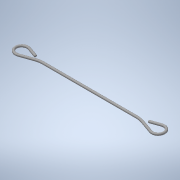
# Autodesk Inventor part: Rebar type 1
Saved by Autodesk Inventor 2021 (Build 250183000, 183)
## iProperties
Company: SDU
Created: 2020-10-29
Part Number: Rebar type 1
Engr Approved By: Approved By
Material: Steel
Description: Description
Document SubType Name: Modeling
Designer: Kling
Engineer: Engineer
Stock Number: Stock number
Density: 7.85 g/cm^3
Appearance: Steel
RM. Dwg. No.: 5674
RM. File Name: N.A.
RM. No.: 4789
Title: Title
Author: Kling
Autodesk Inventor part; units mm, degrees
ref_plane "YZ Plane" through (0, 0, 0) normal (1, 0, 0) x (0, 1, 0)
ref_plane "XZ Plane" through (0, 0, 0) normal (0, 1, 0) x (-1, 0, 0)
ref_plane "XY Plane" through (0, 0, 0) normal (0, 0, 1) x (1, 0, 0)
sketch "Sketch1" plane through (0, 0, 0) normal (0, 0, 1) x (1, 0, 0)
  line L0 (0, 0) -> (-79.8528, 0)
  line L1 (-89.8528, -1.7157) -> (-111.6667, -9.4281)
  arc A0 (-111.6667, 9.4281) -> (-111.6667, -9.4281) centre (-115, 0) ccw
  line L2 (-111.6667, 9.4281) -> (-94.8528, 3.4835)
  arc A1 (-79.8528, 0) -> (-89.8528, -1.7157) centre (-79.8528, -30) ccw
  line L3 (0, 0) -> (0, 44.256) construction
  line L4 (0, 0) -> (79.8528, 0)
  line L5 (89.8528, -1.7157) -> (111.6667, -9.4281)
  arc A2 (111.6667, -9.4281) -> (111.6667, 9.4281) centre (115, 0) ccw
  line L6 (111.6667, 9.4281) -> (94.8528, 3.4835)
  arc A3 (89.8528, -1.7157) -> (79.8528, 0) centre (79.8528, -30) ccw
  point P0 (-85, 0)
  point P1 (85, 0)
  dimension "d0" = 85
  dimension "d1" = 30
  dimension "d2" = 30
  dimension "d3" = 10
  dimension "d4" = 15
  dimension "d5" = 160.529
  dimension "d6" = 160.529
  constraints: 14 end point, 8 point on circle, 8 symmetric about line, 4 centre point, 4 point on line, 4 tangent, 1 horizontal, 1 horizontal alignment, 1 vertical, 2 other
  measures "d0" distance of L0.start point (-85, 0)
  measures "d1" distance of point (-85, 0) A0.centre
  measures "d2" radius of A1
  measures "d3" radius of A0
  measures "d4" horizontal distance of L0.end L2.end
  measures "d5" angle of L0 L1
  measures "d6" angle of L0 L2
sketch "Sketch2" plane through (0, 0, 0) normal (1, 0, 0) x (0, 1, 0)
  circle A0 centre (0, 0) radius 2
  dimension "d7" = 4
  constraints: 1 centre point, 1 coincident
  measures "d7" diameter of A0
sweep "Sweep1" add profiles "Sketch2" path "Sketch1"
chamfer "Chamfer1" distance 1 angle 45 11 edges at (94.1861, 5.3691, 0) (111, 11.3137, 0) (111, -11.3137, 0) (89.1861, -3.6013, 0) (79.8528, -2, 0) (0, -2, 0) (-79.8528, -2, 0) (-89.1861, -3.6013, 0) (-111, -11.3137, 0) (-111, 11.3137, 0) (-94.1861, 5.3691, 0)
equation "\"d6\" = d5"
body "Solid1"
